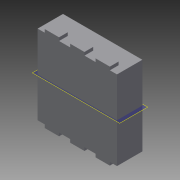
# Autodesk Inventor part: 5050_LED
Saved by Autodesk Inventor 2014 (Build 180170000, 170)
## iProperties
Created: 2013-08-29
Part Number: 5050_LED
Material: Generisch
Document SubType Name: Modeling
Designer: Felix
Density: 1 g/cm^3
Appearance: Vorgabe
Mass: 0.0387168 g
Surface Area: 0.858161 cm^2
Volume: 0.0387168 cm^3
Author: Felix
Autodesk Inventor part; units mm, degrees
ref_plane "YZ Plane" through (0, 0, 0) normal (1, 0, 0) x (0, 1, 0)
ref_plane "XZ Plane" through (0, 0, 0) normal (0, 1, 0) x (-1, 0, 0)
ref_plane "XY Plane" through (0, 0, 0) normal (0, 0, 1) x (1, 0, 0)
sketch "Skizze1" plane through (0, 0, 0) normal (0, 1, 0) x (-1, 0, 0)
  line L0 (0, 0) -> (5, 0)
  line L1 (5, 0) -> (5, 5)
  line L2 (5, 5) -> (0, 5)
  line L3 (0, 5) -> (0, 0)
  dimension "d0" = 5
  dimension "d1" = 5
  constraints: 8 end point, 2 parallel, 1 horizontal, 1 perpendicular
  measures "d0" distance of L2.end L1.end
  measures "d1" distance of L1.end L0.end
extrude "Extrusion1" add sketch "Skizze1" along normal blind 1.6
ref_plane "Arbeitsebene1" through (0, 1.6, 2.5) normal (0, 0, -1) x (-1, 0, 0)
sketch "Skizze2" plane through (-5, 0, 5) normal (0, 0, 1) x (1, 0, 0)
  line L0 (0, 0) -> (5, 0) projected
  line L1 (5, 0) -> (5, 1.6) projected
  line L2 (0, 0) -> (0, 1.6) projected
  line L3 (0.45, 0) -> (1.35, 0)
  line L4 (1.35, 0) -> (1.35, 0.5483)
  line L5 (1.35, 0.5483) -> (0.45, 0.5483)
  line L6 (0.45, 0.5483) -> (0.45, 0)
  line L7 (2.05, 0) -> (2.95, 0)
  line L8 (2.95, 0) -> (2.95, 0.5483)
  line L9 (2.95, 0.5483) -> (2.05, 0.5483)
  line L10 (2.05, 0.5483) -> (2.05, 0)
  line L11 (3.65, 0) -> (4.55, 0)
  line L12 (4.55, 0) -> (4.55, 0.5483)
  line L13 (4.55, 0.5483) -> (3.65, 0.5483)
  line L14 (3.65, 0.5483) -> (3.65, 0)
  line L15 (0.45, 0.5483) -> (0, 0.5483)
  line L16 (4.55, 0.5483) -> (5, 0.5483)
  dimension "d4" = 0.9
  dimension "d5" = 0.9
  dimension "d6" = 0.9
  dimension "d7" = 0.7
  dimension "d8" = 0.7
  constraints: 28 end point, 6 parallel, 5 perpendicular, 5 point on line, 3 collinear, 3 horizontal
  measures "d4" distance of L4.end L5.end
  measures "d5" distance of L8.end L9.end
  measures "d6" distance of L12.end L13.end
  measures "d7" distance between parallel lines of L4 L10
  measures "d8" distance between parallel lines of L14 L8
extrude "Extrusion2" add sketch "Skizze2" along normal blind 0.2 contours L6 L5 L4 L0 | L10 L9 L8 L0 | L14 L13 L12 L0
mirror "Spiegeln1" about plane through (0, 1.6, 2.5) normal (0, 0, -1) of "Extrusion2"
sketch "Skizze3" plane through (0, 1.6, 0) normal (0, 1, 0) x (1, 0, 0)
  circle A0 centre (-2.5, -2.5) radius 2
  dimension "d11" = 4
  constraints: 1 centre point
  measures "d11" diameter of A0
extrude "Extrusion3" cut sketch "Skizze3" against normal blind 0.2
fillet "Rundung1" radius 2 1 edges at (-4.5, 1.4, 2.5)
